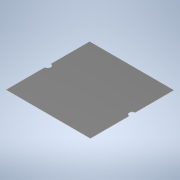
# Autodesk Inventor part: Coverplate Film
Saved by Autodesk Inventor 2022 (Build 260153000, 153)
## iProperties
Created: 2022-02-23
Part Number: Coverplate Film
Material: Thermoplastic Resin
Document SubType Name: Modeling
Designer: Caleb
Density: 1.28 g/cm^3
Appearance: Smooth - Black
Author: Caleb
Autodesk Inventor part; units mm, degrees
ref_plane "YZ Plane" through (0, 0, 0) normal (1, 0, 0) x (0, 1, 0)
ref_plane "XZ Plane" through (0, 0, 0) normal (0, 1, 0) x (-1, 0, 0)
ref_plane "XY Plane" through (0, 0, 0) normal (0, 0, 1) x (1, 0, 0)
sketch "Sketch1" plane through (0, 0, 0) normal (0, 1, 0) x (-1, 0, 0)
  line L0 (-21.7, -21.5) -> (21.7, -21.5)
  line L1 (21.7, -21.5) -> (21.7, 21.5)
  line L2 (21.7, 21.5) -> (-21.7, 21.5)
  line L3 (-21.7, 21.5) -> (-21.7, -21.5)
  line L4 (-21.7, -21.5) -> (21.7, 21.5) construction
  line L5 (21.7, -21.5) -> (-21.7, 21.5) construction
  point P0 (0, 0)
  dimension "d0" = 43
  dimension "d1" = 43.4
  constraints: 12 end point, 2 midpoint, 2 parallel, 1 horizontal, 1 perpendicular
  measures "d0" distance of L0.end L1.end
  measures "d1" distance of L1.end L2.end
extrude "Extrusion1" add sketch "Sketch1" along normal blind 0.08
sketch "Sketch2" plane through (0, 0.08, 0) normal (0, 1, 0) x (1, 0, 0)
  line L0 (-21.7, 21.5) -> (-21.7, -21.5) projected
  arc A0 (-21.7, -1.5) -> (-21.7, 1.5) centre (-21.7, 0) ccw
  line L1 (0, -4.1299) -> (0, 4.8188) construction
  arc A1 (21.7, 1.5) -> (21.7, -1.5) centre (21.7, 0) ccw
  line L2 (21.7, -21.5) -> (21.7, 21.5) projected
  point P0 (0, 0)
  dimension "d5" = 1.5
  constraints: 4 point on circle, 3 symmetric about line, 2 centre point, 2 end point, 2 point on line, 1 midpoint, 1 vertical, 1 other
  measures "d5" radius of A0
extrude "Extrusion2" cut sketch "Sketch2" against normal through all
body "Solid1"
